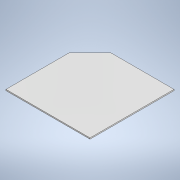
# Autodesk Inventor part: Lid_Clear_Model
Saved by Autodesk Inventor 2022 (Build 260153000, 153)
## iProperties
Created: 2023-02-27
Part Number: Lid_Clear_Model
Material: Generic
Document SubType Name: Modeling
Designer: zarek
Density: 1 g/cm^3
Appearance: Default
Author: zarek
Autodesk Inventor part; units mm, degrees
ref_plane "YZ Plane" through (0, 0, 0) normal (1, 0, 0) x (0, 1, 0)
ref_plane "XZ Plane" through (0, 0, 0) normal (0, 1, 0) x (-1, 0, 0)
ref_plane "XY Plane" through (0, 0, 0) normal (0, 0, 1) x (1, 0, 0)
sketch "Sketch1" plane through (0, 0, 0) normal (0, 1, 0) x (-1, 0, 0)
  line L0 (-90, 90) -> (90, 90)
  line L1 (90, 90) -> (90, -90)
  line L2 (90, -90) -> (-90, -90)
  line L3 (-90, -90) -> (-90, 90)
  line L4 (45.0987, -90) -> (90, -45.0987)
  line L5 (45.0987, -90) -> (108.5987, -90) construction
  point P0 (0, 0)
  point P1 (-90.1, 76.6)
  dimension "d3" = 90
  dimension "d4" = 90
  dimension "d5" = 90
  dimension "d6" = 90
  dimension "d7" = 45
  dimension "d8" = 31.75
  dimension "d9" = 180
  constraints: 12 end point, 2 horizontal, 2 parallel, 2 point on line, 1 equal length, 1 perpendicular
  measures "d3" distance from line of L3 point (0, 0)
  measures "d4" distance from line of L1 point (0, 0)
  measures "d5" distance from line of point (0, 0) L0
  measures "d6" distance from line of L2 point (0, 0)
  measures "d7" angle of L5 L4
  measures "d8" distance from line of L1.end L4
  measures "d9" distance of L2.end L0.start
extrude "Extrusion1" add sketch "Sketch1" along normal blind 2.5 contours L0 L1 L4 L2 L3
body "Solid1"
